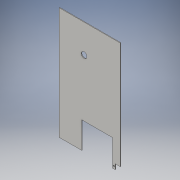
# Autodesk Inventor part: GearboxPlateRev2
Saved by Autodesk Inventor 2016 (Build 200138000, 138)
## iProperties
Created: 2017-01-22
Part Number: GearboxPlateRev2
Material: Generic
Document SubType Name: Modeling
Designer: madsenn
Density: 1 g/cm^3
Appearance: Default
Author: madsenn
Autodesk Inventor part; units mm, degrees
ref_plane "YZ Plane" through (0, 0, 0) normal (1, 0, 0) x (0, 1, 0)
ref_plane "XZ Plane" through (0, 0, 0) normal (0, 1, 0) x (-1, 0, 0)
ref_plane "XY Plane" through (0, 0, 0) normal (0, 0, 1) x (1, 0, 0)
sketch "Sketch1" plane through (0, 0, 0) normal (0, 0, 1) x (1, 0, 0)
  line L0 (-115.6368, 165.4342) -> (189.1632, 165.4342)
  line L1 (189.1632, 165.4342) -> (189.1632, -393.3658)
  line L2 (189.1632, -393.3658) -> (-115.6368, -393.3658)
  line L3 (-115.6368, -393.3658) -> (-115.6368, 165.4342)
  line L4 (151.0632, -393.3658) -> (151.0632, -261.2858)
  line L5 (189.1632, -393.3658) -> (163.5092, -393.3658)
  line L6 (163.5092, -393.3658) -> (163.5092, -367.7118)
  line L7 (163.5092, -367.7118) -> (189.1632, -367.7118)
  line L8 (189.1632, -367.7118) -> (189.1632, -393.3658)
  line L9 (151.0632, -261.2858) -> (-3.064, -261.2858)
  line L10 (-3.064, -261.2858) -> (-3.064, -393.3658)
  circle A0 centre (157.2862, -380.5388) radius 3.5687
  line L11 (189.1632, -317.1658) -> (-115.6368, -317.1658)
  circle A1 centre (9.0264, 24.007) radius 14.2875
  point P0 (0, 0)
  dimension "d0" = 304.8
  dimension "d1" = 558.8
  dimension "d2" = 180.1368
  dimension "d3" = 417.3728
  dimension "d4" = 38.1
  dimension "d5" = 25.654
  dimension "d6" = 25.654
  dimension "d7" = 154.1272
  dimension "d10" = 132.08
  dimension "d11" = 12.446
  dimension "d12" = 6.223
  dimension "d13" = 12.827
  dimension "d14" = 7.1374
  dimension "d15" = 76.2
  dimension "d16" = 28.575
  constraints: 24 end point, 4 parallel, 4 perpendicular, 4 point on line, 3 horizontal, 2 centre point, 2 coincident, 1 vertical
  measures "d0" distance of L0.start L0.end
  measures "d1" distance of L2.end L0.start
  measures "d2" distance from line of point (9.026, 24.007) L1
  measures "d3" distance from line of L2 point (9.026, 24.007)
  measures "d4" distance between parallel lines of L1 L4
  measures "d5" distance of L6.end L7.end
  measures "d6" distance between parallel lines of L2 L7
  measures "d7" distance of L4.end L9.end
  measures "d10" distance of L9.end L10.end
  measures "d11" distance between parallel lines of L6 L4
  measures "d12" distance from line of L6 point (157.286, -380.539)
  measures "d13" distance from line of L2 point (157.286, -380.539)
  measures "d14" diameter of A0
  measures "d15" distance between parallel lines of L2 L11
  measures "d16" diameter of A1
extrude "Extrusion1" add sketch "Sketch1" along normal blind 3.175 contours L0 L1 L11 L4 L9 L10 L3 | L11 L10 L2 L3 | L1 L7 L6 L2 L4 L11
body "Solid1"
